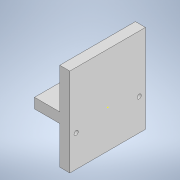
# Autodesk Inventor part: 25_Laser_adapter
Saved by Autodesk Inventor 2022.2 (Build 262287010, 287A)
## iProperties
Created: 2022-05-02
Part Number: 25_Laser_adapter
Material: Generisch
Document SubType Name: Modeling
Designer: MXBD
Density: 1 g/cm^3
Appearance: Vorgabe
Author: MXBD
Autodesk Inventor part; units mm, degrees
ref_plane "YZ Plane" through (0, 0, 0) normal (1, 0, 0) x (0, 1, 0)
ref_plane "XZ Plane" through (0, 0, 0) normal (0, 1, 0) x (-1, 0, 0)
ref_plane "XY Plane" through (0, 0, 0) normal (0, 0, 1) x (1, 0, 0)
sketch "Skizze1" plane through (0, 0, 0) normal (0, 0, 1) x (1, 0, 0)
  line L0 (0, 54) -> (0, -44) projected
  line L1 (-33.6, 0) -> (5.6, 0) projected
  line L2 (-8, 40) -> (0, 40)
  line L3 (0, 40) -> (0, -30)
  line L4 (0, -30) -> (-8, -30)
  line L5 (-8, -30) -> (-8, 0)
  line L6 (-8, 0) -> (-28, 0)
  line L7 (-28, 0) -> (-28, 8)
  line L8 (-28, 8) -> (-8, 8)
  line L9 (-8, 8) -> (-8, 40)
  point P0 (0, 0)
  dimension "d0" = 70
  dimension "d1" = 8
  dimension "d2" = 20
  dimension "d3" = 8
  dimension "d4" = 40
  constraints: 16 end point, 5 point on line, 4 perpendicular, 1 horizontal, 1 vertical
  measures "d0" distance between parallel lines of L4 L2
  measures "d1" distance between parallel lines of L9 L3
  measures "d2" distance between parallel lines of L7 L9
  measures "d3" distance of L6.end L7.end
  measures "d4" distance between parallel lines of L1 L2
extrude "Extrusion1" add sketch "Skizze1" along normal mid plane 60
sketch "Skizze2" plane through (0, -30, 30) normal (1, 0, 0) x (0, 0, -1)
  point P0 (30, 30)
sketch "Skizze3" plane through (0, -30, 30) normal (1, 0, 0) x (0, 0, -1)
  line L0 (-12, 30) -> (72, 30) projected
  line L1 (30, -14) -> (30, 84) projected
  line L2 (60, 70) -> (0, 70) projected
  point P0 (30, 30)
  point P1 (5, 25)
  point P2 (55, 25)
  dimension "d7" = 50
  dimension "d8" = 45
  constraints: 1 symmetric about line
  measures "d7" distance of point (55, 25) point (5, 25)
  measures "d8" distance from line of point (55, 25) L2
hole "Bohrung1" at (0, -5, 25) at (0, -5, -25) direction (-1, 0, 0) diameter 3.4 end through all clearance for "Inbusschraube ISO 4762" size "M3" standard "ISO"
